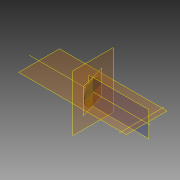
# Autodesk Inventor part: butterfly
Saved by Autodesk Inventor 2015 (Build 190159000, 159)
## iProperties
Created: 2015-09-04
Part Number: butterfly
Material: Brass, Soft Yellow
Description: insert part description/title
Document SubType Name: Modeling
Designer: francis
Density: 8.47 g/cm^3
Appearance: Brass - Satin
Part Category: insert part category here and press enter to fill value
Author: francis
Autodesk Inventor part; units mm, degrees
ref_plane "YZ Plane" through (0, 0, 0) normal (1, 0, 0) x (0, 1, 0)
ref_plane "XY Plane" through (0, 0, 0) normal (0, 0, 1) x (1, 0, 0)
ref_plane "Work Plane1" through (0, 0, 0) normal (0, 0, 1) x (1, 0, 0)
sketch "Sketch1" plane through (0, 0, 0) normal (0, 0, 1) x (1, 0, 0)
  line L0 (-58.0302, -14) -> (-60.5225, -14) construction
  line L1 (-54.7493, -17.6642) -> (-59.4824, 0)
  line L2 (-65.1814, 17.4053) -> (-55.7152, -17.923)
  line L3 (-59.4824, 0) -> (-60.5176, 0) construction
  line L4 (-144, 0) -> (-60.5176, 0) construction
  line L5 (-47.8265, 0) -> (-82.556, 0) construction
  line L6 (-64.2155, 17.6642) -> (-65.1814, 17.4053)
  line L7 (-55.7152, -17.923) -> (-54.7493, -17.6642)
  line L8 (-59.4824, 0) -> (-64.2155, 17.6642)
  line L9 (-60.5176, 0) -> (24, 0) construction
  line L10 (-144, 0) -> (24, 0)
  line L11 (-60, 54.8295) -> (-60, -83.9771)
  point P0 (0, 0)
  point P1 (-60, 0)
  dimension "d2" = 1
  dimension "d28" = 17.6642
  dimension "d29" = 15
  constraints: 24 end point, 10 point on line, 3 horizontal, 3 midpoint, 3 perpendicular, 2 parallel, 1 collinear, 1 vertical, 6 other
  measures "d2" distance between parallel lines of L2 L1
  measures "d28" distance from line of L4 L6.start
  measures "d29" angle of L11 L2
extrude "Extrusion1" add sketch "Sketch1" along normal blind 30 and the other way blind 30
ref_plane "Work Plane2" through (-60, 0, -16) normal (1, 0, 0) x (0, 0, -1)
sketch "Sketch2" plane through (-60, 0, -16) normal (1, 0, 0) x (0, 0, -1)
  circle A0 centre (-16, 0) radius 17.5
  dimension "d26" = 35
  constraints: 1 centre point, 1 coincident
  measures "d26" diameter of A0
extrude "Extrusion2" cut sketch "Sketch2" along normal mid plane 30 keep common part
sketch "Sketch5" plane through (-60, 0, -16) normal (1, 0, 0) x (0, 0, -1)
  circle A0 centre (-16, 0) radius 14
  dimension "d30" = 28
  constraints: 1 centre point, 1 coincident
  measures "d30" diameter of A0
extrude "Extrusion4" cut sketch "Sketch5" along normal mid plane 10 keep common part
sketch "Sketch7" plane through (-59.4824, 0, 0) normal (0.9659, 0.2588, 0) x (0, 0, -1)
  line L0 (-33.8, 0.134) -> (-42.2, 0.134) construction
  line L1 (-86, 0.134) -> (89, 0.134) construction
  line L2 (-86, 0.134) -> (89, 0.134) construction
  circle A0 centre (7.5, 0.134) radius 1.5 construction
  circle A1 centre (-7.5, 0.134) radius 1.5 construction
  line L3 (0, -21.4266) -> (0, 20.7932) construction
  point P0 (0, -15.3952)
  dimension "d34" = 3
  dimension "d35" = 7.5
  dimension "d36" = 7.5
  constraints: 6 end point, 3 horizontal, 2 centre point, 2 point on line, 1 equal radius, 6 other
  measures "d34" diameter of A1
  measures "d35" distance from line of L3 A0.centre
  measures "d36" distance from line of A1.centre L3
hole "Hole2" at (-59.517, 0.1294, -7.5) at (-59.517, 0.1294, 7.5) direction (-0.9659, -0.2588, 0) diameter 3 end through all
body "Solid1"
